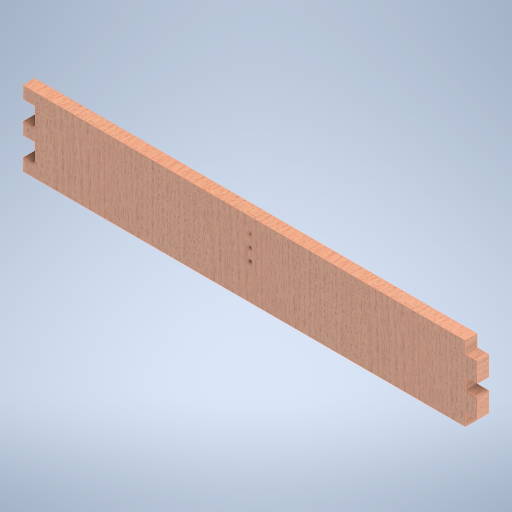
# Autodesk Inventor part: Bumper wood
Saved by Autodesk Inventor 2023 (Build 270158000, 158)
## iProperties
Created: 2023-11-22
Part Number: Bumper wood
Material: Wood (Oak)
Document SubType Name: Modeling
Designer: adamarnold
Density: 0.76 g/cm^3
Appearance: White Oak - Natural Medium Gloss
Author: adamarnold
Autodesk Inventor part; units mm, degrees
ref_plane "YZ Plane" through (0, 0, 0) normal (1, 0, 0) x (0, 1, 0)
ref_plane "XZ Plane" through (0, 0, 0) normal (0, 1, 0) x (-1, 0, 0)
ref_plane "XY Plane" through (0, 0, 0) normal (0, 0, 1) x (1, 0, 0)
sketch "Sketch1" plane through (0, 0, 0) normal (0, 0, 1) x (1, 0, 0)
  line L0 (0, 0) -> (-733.425, 0)
  line L1 (-733.425, 0) -> (-733.425, 120.65)
  line L2 (-733.425, 120.65) -> (0, 120.65)
  line L3 (0, 120.65) -> (0, 0)
  dimension "d0" = 733.425
  dimension "d1" = 120.65
  constraints: 8 end point, 2 parallel, 1 horizontal, 1 perpendicular
  measures "d0" distance of L1.end L2.end
  measures "d1" distance of L0.end L1.end
extrude "Extrusion1" add sketch "Sketch1" along normal blind 19.05
sketch "Sketch2" plane through (0, 0, 19.05) normal (0, 0, 1) x (1, 0, 0)
  line L0 (0, 120.65) -> (-733.425, 120.65) projected
  line L1 (0, 120.65) -> (-19.304, 120.65)
  line L2 (-19.304, 120.65) -> (-19.304, 101.346)
  line L3 (-19.304, 101.346) -> (0, 101.346)
  line L4 (0, 101.346) -> (0, 120.65)
  line L5 (0, 0) -> (-19.304, 0)
  line L6 (-19.304, 0) -> (-19.304, 19.304)
  line L7 (-19.304, 19.304) -> (0, 19.304)
  line L8 (0, 19.304) -> (0, 0)
  line L9 (0, 0) -> (0, 120.65) projected
  line L10 (0, 60.325) -> (-19.304, 60.325)
  line L11 (0, 69.977) -> (-19.304, 69.977)
  line L12 (0, 50.673) -> (-19.304, 50.673)
  line L13 (-19.304, 69.977) -> (-19.304, 50.673)
  line L14 (0, 69.977) -> (0, 50.673)
  line L15 (-733.425, 120.65) -> (-733.425, 0) projected
  line L16 (-733.425, 120.65) -> (-733.425, 101.346)
  line L17 (-733.425, 101.346) -> (-714.121, 101.346)
  line L18 (-714.121, 101.346) -> (-733.425, 101.346)
  line L19 (-733.425, 101.346) -> (-733.425, 69.977)
  line L20 (-733.425, 69.977) -> (-714.121, 69.977)
  line L21 (-714.121, 69.977) -> (-714.121, 101.346)
  line L22 (-733.425, 60.325) -> (-720.7714, 60.325)
  line L23 (-733.425, 0) -> (-733.425, 120.65)
  line L24 (-733.425, 0) -> (-733.425, 19.304)
  line L25 (-733.425, 19.304) -> (-714.121, 19.304)
  line L26 (-714.121, 19.304) -> (-733.425, 19.304)
  line L27 (-733.425, 19.304) -> (-733.425, 50.673)
  line L28 (-733.425, 50.673) -> (-714.121, 50.673)
  line L29 (-714.121, 50.673) -> (-714.121, 19.304)
  dimension "d4" = 19.304
  dimension "d5" = 19.304
  dimension "d6" = 19.304
  dimension "d7" = 19.304
  dimension "d8" = 19.304
  dimension "d9" = 9.652
  dimension "d10" = 9.652
  dimension "d14" = 19.304
  dimension "d15" = 19.304
  dimension "d16" = 31.369
  constraints: 54 end point, 9 parallel, 7 symmetric about line, 5 horizontal, 4 perpendicular, 4 point on line, 2 midpoint, 1 vertical
  measures "d4" distance of L3.end L2.end
  measures "d5" distance of L2.end L1.end
  measures "d6" distance of L6.end L7.end
  measures "d7" distance of L5.end L6.end
  measures "d8" distance of L10.start L10.end
  measures "d9" distance between parallel lines of L10 L11
  measures "d10" distance between parallel lines of L10 L12
  measures "d14" distance of L0.end L16.end
  measures "d15" distance of L16.end L17.end
  measures "d16" distance of L19.end L18.end
extrude "Extrusion2" cut sketch "Sketch2" against normal through all
sketch "Sketch3" plane through (0, 0, 19.05) normal (0, 0, 1) x (1, 0, 0)
  line L0 (-733.425, 120.65) -> (-733.425, 101.346) projected
  line L1 (-366.7125, 120.65) -> (-366.7125, 18.5529)
  line L2 (-366.7125, 95.25) -> (-285.5796, 95.25)
  line L3 (-366.7125, 76.2) -> (-319.7387, 76.2)
  line L4 (-366.7125, 57.15) -> (-319.7387, 57.15)
  line L5 (-714.121, 101.346) -> (-714.121, 69.977) projected
  line L6 (-714.121, 101.346) -> (-714.121, 120.65)
  point P0 (0, 0)
  point P1 (-326.1461, 95.25)
  point P2 (-714.121, 110.998)
  dimension "d30" = 347.4085
  constraints: 10 end point, 3 horizontal, 3 point on line, 2 midpoint, 1 vertical
  measures "d30" distance from line of L1 point (-714.121, 110.998)
hole "Hole1" at (-366.7125, 95.25, 19.05) at (-366.7125, 76.2, 19.05) at (-366.7125, 57.15, 19.05) direction (0, 0, -1) diameter 6.35 end through all
body "Solid1"
